Autodesk Fusion 360 part; units mm, degrees
(part 2 of 2)
  arc A148 (4.5, 28.5) -> (3.5, 27.5) centre (4.5, 27.5) ccw
  line L175 (1.7929, 170.8284) -> (15.7929, 156.8284)
  line L176 (17.5, 157.5355) -> (17.5, 159.833)
  line L177 (17.2071, 160.5402) -> (3.2071, 174.5402)
  line L178 (1.5, 173.833) -> (1.5, 171.5355)
  arc A149 (1.5, 171.5355) -> (1.7929, 170.8284) centre (2.5, 171.5355) ccw
  arc A150 (3.2071, 174.5402) -> (1.5, 173.833) centre (2.5, 173.833) ccw
  arc A151 (17.5, 159.833) -> (17.2071, 160.5402) centre (16.5, 159.833) ccw
  arc A152 (15.7929, 156.8284) -> (17.5, 157.5355) centre (16.5, 157.5355) ccw
  line L179 (2.3284, 9.7071) -> (8.7929, 16.1716)
  line L180 (10.5, 15.4645) -> (10.5, 9)
  line L181 (9.5, 8) -> (3.0355, 8)
  arc A153 (2.3284, 9.7071) -> (3.0355, 8) centre (3.0355, 9) ccw
  arc A154 (9.5, 8) -> (10.5, 9) centre (9.5, 9) ccw
  arc A155 (10.5, 15.4645) -> (8.7929, 16.1716) centre (9.5, 15.4645) ccw
  arc A156 (-23.9472, 177.9837) -> (-22.7624, 177.0888) centre (-22.951, 178.0708) ccw
  arc A157 (-24.2217, 193.0163) -> (-25.1674, 191.9304) centre (-24.1712, 192.0175) ccw
  arc A158 (19.6886, 185.2415) -> (20.4962, 186.3107) centre (19.5, 186.2235) ccw
  arc A159 (19.7989, 194.2803) -> (18.7522, 195.1918) centre (18.8028, 194.1931) ccw
  line L182 (-22.5614, 176.267) -> (-23.6581, 177.3637)
  point P0 (19.8308, 195.2464)
  point P1 (-25.2578, 192.9638)
  point P2 (-23.8633, 177.0247)
  point P3 (-87.3104, 78.3815)
  dimension "d191" = 1
  dimension "d192" = 7.5
  dimension "d193" = 1.5
  dimension "d194" = 27
  dimension "d195" = 24
  dimension "d196" = 35
  dimension "d199" = 1.5
  dimension "d200" = 2.5
  dimension "d201" = 5
  dimension "d202" = 2
  dimension "d203" = 0.4
  dimension "d204" = 1
  dimension "d205" = 30
  dimension "d206" = 0.2
  dimension "d207" = 5
  dimension "d209" = 2
  dimension "d210" = 3
  dimension "d211" = 1
  dimension "d212" = 20
  dimension "d214" = 20
  dimension "d215" = 180
  dimension "d216" = 90
  dimension "d217" = 5
  dimension "d225" = 2
  dimension "d228" = 2
  dimension "d229" = 1.5
  dimension "d230" = 45
  dimension "d233" = 10
  dimension "d234" = 12.7
  dimension "d235" = 3
  dimension "d237" = 20
  dimension "d240" = 2
  dimension "d241" = 2
  dimension "d242" = 2
  dimension "d243" = 16
  dimension "d245" = 45
  dimension "d246" = 20
  dimension "d247" = 20
  dimension "d249" = 90
  dimension "d250" = 5
  dimension "d251" = 5
  dimension "d252" = 3
  dimension "d253" = 5
  dimension "d287" = 20
  dimension "d288" = 2
  dimension "d296" = 5
  dimension "d297" = 2
  dimension "d299" = 60
  dimension "d300" = 2.5
  dimension "d301" = 1
  dimension "d303" = 360
  dimension "d306" = 7.5
  dimension "d307" = 5
  dimension "d309" = 30
  dimension "d310" = 1
  dimension "d311" = 20
  dimension "d312" = 3
  dimension "d313" = 1
  dimension "d314" = 3
  dimension "d315" = 1.5
  dimension "d316" = 1.5
  dimension "d317" = 1
  dimension "d318" = 1.5
  dimension "d319" = 3
  dimension "d320" = 1.5
  dimension "d321" = 1.5
  dimension "d322" = 3
  dimension "d323" = 1.5
  dimension "d324" = 1
  dimension "d325" = 1
  dimension "d326" = 3
  dimension "d327" = 1.5
  dimension "d328" = 1.5
  dimension "d329" = 3
  dimension "d330" = 3
  dimension "d331" = 3
  dimension "d332" = 3
  dimension "d333" = 1.5
  dimension "d334" = 1.5
  dimension "d335" = 1.5
  dimension "d336" = 1.5
  dimension "d337" = 1.5
  dimension "d338" = 1.5
  dimension "d339" = 1.5
  dimension "d340" = 1.5
  dimension "d341" = 1
  dimension "d342" = 1
  dimension "d343" = 3
  dimension "d344" = 1.5
  dimension "d345" = 1.5
  dimension "d346" = 1
  dimension "d347" = 1.5
  dimension "d348" = 3
  dimension "d349" = 3
  dimension "d350" = 1.5
  dimension "d351" = 1.5
  dimension "d352" = 3
  dimension "d353" = 1
  dimension "d354" = 3
  dimension "d355" = 3
  dimension "d356" = 1
  dimension "d357" = 1
  dimension "d358" = 1.5
  dimension "d359" = 45
  dimension "d360" = 1.5
  dimension "d361" = 3
  dimension "d362" = 1.5
  dimension "d363" = 1.5
  dimension "d364" = 3
  dimension "d365" = 1.5
  dimension "d366" = 1
  dimension "d369" = -20
  dimension "d370" = 0
  dimension "d371" = 1.5
  dimension "d372" = 3
  dimension "d373" = 1.5
  dimension "d374" = 1
  dimension "d375" = 1.5
  dimension "d376" = 3
  dimension "d377" = 3
  dimension "d378" = 3
  dimension "d379" = 1
  dimension "d380" = 1
  dimension "d381" = 3
  dimension "d382" = 3
  dimension "d383" = 3
  dimension "d390" = 1
  dimension "d391" = 100
  dimension "d392" = 14
  dimension "d393" = 8
  dimension "d394" = 20
  constraint vertical L0
  constraint perpendicular L0 L1
  constraint perpendicular L1 L2
  constraint perpendicular L2 L3
  constraint perpendicular L3 L4
  constraint perpendicular L4 L5
  constraint perpendicular L5 L6
  constraint perpendicular L0 L7
  constraint perpendicular L7 L8
  constraint perpendicular L0 L9
  constraint perpendicular L7 L10
  constraint perpendicular L0 L11
  constraint symmetric L2 L4 L12
  constraint symmetric L0 L6 L12
  constraint collinear origin L0.start L10.end
  constraint collinear origin L6.end L7.end
  constraint coincident L1 L5.end
  constraint perpendicular L1 L14
  constraint perpendicular L14 L15
  constraint tangent L14 A1
  constraint tangent L16 A1
  constraint tangent L14 A2
  constraint tangent L15 A2
  constraint equal A1 A2
  constraint tangent L15 A3
  constraint parallel L5 L17
  constraint perpendicular L5 L18
  constraint parallel L17 L20
  constraint perpendicular L17 L31
  constraint tangent L19 A4
  constraint tangent L17 A4
  constraint tangent L19 A5
  constraint tangent L20 A5
  constraint tangent L20 A6
  constraint tangent A6 L31
  constraint equal A5 A6
  constraint perpendicular L5 L21
  constraint tangent A4 L21
  constraint tangent L18 A7
  constraint perpendicular L13 L22
  constraint tangent L22 A7
  constraint horizontal L23
  constraint tangent A7 L23
  constraint coincident L6 L18.end
  constraint concentric A0 A8
  constraint coincident A8 L24.start
  constraint tangent A8 L24
  constraint perpendicular L24 L25
  constraint perpendicular L24 L27
  constraint tangent A0 L29
  constraint collinear L31 L32
  constraint perpendicular L22 L33
  constraint coincident origin L30
  constraint tangent L32 A9
  constraint tangent L33 A9
  constraint tangent L33 A10
  constraint tangent L30 A11
  constraint tangent L31 A11
  constraint concentric A0 A12
  constraint concentric A8 A13
  constraint vertical L36
  constraint parallel L29 L35
  constraint tangent L34 A14
  constraint tangent L36 A14
  constraint tangent L35 A15
  constraint tangent L36 A15
  constraint equal A14 A15
  constraint perpendicular L29 L37
  constraint tangent L29 A16
  constraint tangent L37 A17
  constraint tangent L28 A17
  constraint symmetric L24 P1 P2
  constraint vertical L38
  constraint tangent A3 L38
  constraint tangent A0 L39
  constraint tangent L37 A18
  constraint coincident L28 A17.start
  constraint perpendicular L38 L40
  constraint perpendicular L40 L41
  constraint tangent L40 A19
  constraint tangent L41 A19
  constraint coincident A20.centre A44.centre
  constraint coincident L32 A18.start
  constraint coincident A7.centre A21.centre
  constraint tangent L32 A21
  constraint coincident L32 A21.start
  constraint coincident L32.end A18.start
  constraint tangent L32 A18
  constraint coincident A0.centre A8.centre
  constraint tangent A22 A23
  constraint tangent L34 A23
  constraint tangent A22 A24
  constraint tangent L35 A24
  constraint equal A23 A24
  constraint horizontal L46
  constraint symmetric L43 L44 L46
  constraint parallel L43 L45
  constraint tangent L44 A27
  constraint tangent A25 A27
  constraint tangent A26 A28
  constraint tangent L44 A28
  constraint equal A27 A28
  constraint coincident P3 L43
  constraint coincident P3 A25
  constraint tangent A25 A29
  constraint tangent L43 A29
  constraint equal A27 A29
  constraint tangent A26 A30
  constraint tangent L43 A30
  constraint equal A27 A30
  constraint vertical L51
  constraint tangent L51 A44
  constraint tangent A43 A44
  constraint tangent A20 A43
  constraint tangent L51 A45
  constraint tangent L30 A45
  constraint collinear A20.centre A43.centre L52.end
  constraint perpendicular L12 L30
  constraint coincident L6.end L7
  constraint tangent L22 A46
  constraint tangent L7 A46
  constraint equal A9 A10
  constraint coincident A10.end A20.end
  constraint tangent A10 A20
  constraint horizontal L53
  constraint collinear A20.centre A10.end L53.end
  constraint midpoint L36 L54.start
  constraint coincident L39 L54.end
  constraint perpendicular L39 L54
  constraint coincident L34 L55.end
  constraint vertical L55
  constraint coincident L39 L56.end
  constraint perpendicular L39 L56
  constraint parallel L55 L57
  constraint coincident L34 L57.end
  constraint coincident L39 L58.end
  constraint perpendicular L39 L58
  constraint perpendicular L39 L60
  constraint vertical L61
  constraint tangent L59 A47
  constraint tangent L60 A47
  constraint tangent L60 A48
  constraint tangent L61 A48
  constraint equal A47 A48
  constraint tangent L59 A49
  constraint tangent L61 A49
  constraint equal A47 A49
  constraint parallel L39 L59
  constraint vertical L62
  constraint perpendicular L39 L64
  constraint perpendicular L63 L64
  constraint tangent L62 A50
  constraint tangent L64 A50
  constraint tangent L62 A51
  constraint tangent L63 A51
  constraint equal A50 A51
  constraint tangent L63 A52
  constraint tangent L64 A52
  constraint equal A50 A52
  constraint coincident L34 L65.start
  constraint coincident L39 L65.end
  constraint coincident L54 L65.start
  constraint parallel L12 L65
  constraint coincident L34 L66.end
  constraint perpendicular L34 L66
  constraint parallel L57 L69
  constraint perpendicular L39 L67
  constraint perpendicular L67 L68
  constraint tangent L67 A53
  constraint tangent L69 A53
  constraint tangent L68 A54
  constraint tangent L69 A54
  constraint equal A53 A54
  constraint tangent L67 A55
  constraint tangent L68 A55
  constraint equal A53 A55
  constraint perpendicular L39 L71
  constraint perpendicular L70 L71
  constraint parallel L57 L72
  constraint tangent L70 A56
  constraint tangent L72 A56
  constraint tangent L70 A57
  constraint tangent L71 A57
  constraint equal A56 A57
  constraint tangent L71 A58
  constraint tangent L72 A58
  constraint equal A56 A58
  constraint coincident L39 L73.end
  constraint vertical L73
  constraint coincident L34 L74.end
  constraint perpendicular L34 L74
  constraint coincident L40 L75.end
  constraint perpendicular L40 L75
  constraint perpendicular L78 L79
  constraint vertical L81
  constraint perpendicular L85 L87
  constraint perpendicular L83 L84
  constraint perpendicular L79 L80
  constraint perpendicular L34 L84
  constraint perpendicular L39 L87
  constraint perpendicular L39 L80
  constraint perpendicular L77 L78
  constraint parallel L65 L82
  constraint parallel L65 L86
  constraint parallel L73 L76
  constraint tangent L85 A59
  constraint tangent L87 A59
  constraint tangent L86 A60
  constraint tangent L87 A60
  constraint equal A59 A60
  constraint tangent L85 A61
  constraint tangent L86 A61
  constraint equal A59 A61
  constraint tangent L82 A62
  constraint tangent L84 A62
  constraint equal A59 A62
  constraint tangent L82 A63
  constraint tangent L83 A63
  constraint equal A59 A63
  constraint tangent L83 A64
  constraint tangent L84 A64
  constraint equal A59 A64
  constraint tangent L79 A65
  constraint tangent L80 A65
  constraint equal A59 A65
  constraint tangent L79 A66
  constraint tangent L81 A66
  constraint equal A59 A66
  constraint tangent L80 A67
  constraint tangent L81 A67
  constraint equal A59 A67
  constraint tangent L76 A68
  constraint tangent L77 A68
  constraint equal A59 A68
  constraint tangent L76 A69
  constraint tangent L78 A69
  constraint equal A59 A69
  constraint tangent L77 A70
  constraint tangent L78 A70
  constraint equal A59 A70
  constraint parallel L40 L90
  constraint parallel L74 L88
  constraint parallel L75 L89
  constraint tangent L90 A71
  constraint tangent L88 A71
  constraint tangent L89 A72
  constraint tangent L90 A72
  constraint equal A71 A72
  constraint tangent L88 A73
  constraint tangent L89 A73
  constraint equal A71 A73
  constraint parallel L75 L91
  constraint parallel L40 L93
  constraint parallel L34 L92
  constraint tangent L91 A74
  constraint tangent L93 A74
  constraint tangent L91 A75
  constraint tangent L92 A75
  constraint equal A74 A75
  constraint tangent L92 A76
  constraint tangent L93 A76
  constraint equal A74 A76
  constraint symmetric L46 L59.end L100.end
  constraint symmetric L46 L60.start L102.start
  constraint symmetric L46 A47 A85
  constraint symmetric L46 L60.end A84.start
  constraint symmetric L46 L61.start L101.start
  constraint symmetric L46 A48 A84
  constraint symmetric L46 L59.start A83.end
  constraint symmetric L46 L61.end A83.start
  constraint symmetric L46 A49 A83
  constraint symmetric L46 L62.start A86.end
  constraint symmetric L46 L64.end A86.start
  constraint symmetric L46 A50 A86
  constraint symmetric L46 L62.end L103.end
  constraint symmetric L46 L63.start L105.start
  constraint symmetric L46 A51 A88
  constraint symmetric L46 L63.end L105.end
  constraint symmetric L46 L64.start L104.start
  constraint symmetric L46 A52 A87
  constraint symmetric L46 L67.start A81.start
  constraint symmetric L46 L69.end L97.end
  constraint symmetric L46 A53 A81
  constraint symmetric L46 L68.end A80.end
  constraint symmetric L46 L69.start A80.start
  constraint symmetric L46 A54 A80
  constraint symmetric L46 L67.end L98.end
  constraint symmetric L46 L68.start L99.start
  constraint symmetric L46 A55 A82
  constraint symmetric L46 L70.start L94.start
  constraint symmetric L46 L72.end L96.end
  constraint symmetric L46 A56 A78
  constraint symmetric L46 L70.end L94.end
  constraint symmetric L46 L71.start L95.start
  constraint symmetric L46 A57 A79
  constraint symmetric L46 L71.end L95.end
  constraint symmetric L46 L72.start A77.end
  constraint symmetric L46 A58 A77
  constraint symmetric L46 L85.start A89.start
  constraint symmetric L46 L87.end A89.end
  constraint symmetric L46 A59 A89
  constraint symmetric L46 L86.end L108.end
  constraint symmetric L46 L87.start L107.start
  constraint symmetric L46 A60 A90
  constraint symmetric L46 L85.end L106.end
  constraint symmetric L46 L86.start L108.start
  constraint symmetric L46 A61 A91
  constraint symmetric L46 L82.start A92.end
  constraint symmetric L46 L84.end A92.start
  constraint symmetric L46 A62 A92
  constraint symmetric L46 L82.end L109.end
  constraint symmetric L46 L83.start L111.start
  constraint symmetric L46 A63 A94
  constraint symmetric L46 L83.end A93.start
  constraint symmetric L46 L84.start L110.start
  constraint symmetric L46 A64 A93
  constraint symmetric L46 L79.end L112.end
  constraint symmetric L46 L80.start L114.start
  constraint symmetric L46 A65 A97
  constraint symmetric L46 L79.start L112.start
  constraint symmetric L46 L81.end A95.start
  constraint symmetric L46 A66 A95
  constraint symmetric L46 L80.end A96.start
  constraint symmetric L46 L81.start L113.start
  constraint symmetric L46 A67 A96
  constraint symmetric L46 L76.end L115.end
  constraint symmetric L46 L77.start L117.start
  constraint symmetric L46 A68 A99
  constraint symmetric L46 L76.start L115.start
  constraint symmetric L46 L78.end L116.end
  constraint symmetric L46 A69 A98
  constraint symmetric L46 L77.end L117.end
  constraint symmetric L46 L78.start L116.start
  constraint symmetric L46 A70 A100
  constraint coincident L29 L118.start
  constraint coincident L35 L118.end
  constraint parallel L116 L118
  constraint perpendicular L119 L120
  constraint perpendicular L35 L119
  constraint tangent L119 A101
  constraint tangent L120 A101
  constraint tangent L119 A102
  constraint tangent L121 A102
  constraint equal A101 A102
  constraint tangent L120 A103
  constraint tangent L121 A103
  constraint equal A101 A103
  constraint symmetric L115 L118 L121
  constraint vertical L122
  constraint parallel L28 L123
  constraint parallel L121 L124
  constraint tangent L124 A104
  constraint tangent L123 A104
  constraint tangent L122 A105
  constraint tangent L124 A105
  constraint tangent L122 A106
  constraint tangent L123 A106
  constraint equal A105 A106
  constraint coincident L32 L125.end
  constraint perpendicular L32 L125
  constraint coincident L36 L126.end
  constraint coincident L32 L127.end
  constraint perpendicular L32 L127
  constraint coincident L36 L128.end
  constraint coincident L32 L129.end
  constraint perpendicular L32 L129
  constraint coincident L36 L130.end
  constraint parallel L126 L128
  constraint parallel L128 L130
  constraint coincident L32 L131.end
  constraint perpendicular L32 L131
  constraint parallel L130 L132
  constraint parallel L126 L136
  constraint parallel L126 L134
  constraint perpendicular L133 L135
  constraint perpendicular L137 L138
  constraint perpendicular L32 L138
  constraint perpendicular L36 L135
  constraint tangent L133 A107
  constraint tangent L134 A107
  constraint tangent L133 A108
  constraint tangent L135 A108
  constraint equal A107 A108
  constraint tangent L134 A109
  constraint tangent L135 A109
  constraint equal A107 A109
  constraint tangent L136 A110
  constraint tangent L137 A110
  constraint equal A107 A110
  constraint tangent L136 A111
  constraint tangent L138 A111
  constraint equal A107 A111
  constraint tangent L137 A112
  constraint tangent L138 A112
  constraint equal A107 A112
  constraint parallel L131 L151
  constraint perpendicular L151 L153
  constraint parallel L132 L152
  constraint tangent L151 A125
  constraint tangent L153 A125
  constraint tangent L152 A126
  constraint tangent L153 A126
  constraint equal A125 A126
  constraint tangent L151 A127
  constraint tangent L152 A127
  constraint equal A125 A127
  constraint symmetric L125 L133.end L154.end
  constraint symmetric L125 L134.start L156.start
  constraint symmetric L125 A107 A129
  constraint symmetric L125 L133.start L154.start
  constraint symmetric L125 L135.end A128.start
  constraint symmetric L125 A108 A128
  constraint symmetric L125 L134.end L156.end
  constraint symmetric L125 L135.start L155.start
  constraint symmetric L125 A109 A130
  constraint symmetric L125 L136.end L157.end
  constraint symmetric L125 L137.start A131.start
  constraint symmetric L125 A110 A131
  constraint symmetric L125 L136.start L157.start
  constraint symmetric L125 L138.end L159.end
  constraint symmetric L125 A111 A133
  constraint symmetric L125 L137.end L158.end
  constraint symmetric L125 L138.start A132.start
  constraint symmetric L125 A112 A132
  constraint symmetric L125 A113.start L160.start
  constraint symmetric L125 A113.end A134.start
  constraint symmetric L125 A113 A134
  constraint symmetric L125 A114.start A136.end
  constraint symmetric L125 A114.end L161.end
  constraint symmetric L125 A114 A136
  constraint symmetric L125 L140.start A135.end
  constraint symmetric L125 A115.end L160.end
  constraint symmetric L125 A115 A135
  constraint symmetric L125 L142.start A137.start
  constraint symmetric L125 L142.end L164.end
  constraint symmetric L125 A116.start L163.end
  constraint symmetric L125 A116 A137
  constraint symmetric L125 L143.start L163.start
  constraint symmetric L125 L144.start A138.start
  constraint symmetric L125 L144.end L165.end
  constraint symmetric L125 A117 A139
  constraint symmetric L125 A118 A138
  constraint symmetric L125 A119.start L167.start
  constraint symmetric L125 A119.end L166.end
  constraint symmetric L125 A119 A142
  constraint symmetric L125 A120.start A140.end
  constraint symmetric L125 A120.end A140.start
  constraint symmetric L125 A120 A140
  constraint symmetric L125 L146.start A141.end
  constraint symmetric L125 A121.end A141.start
  constraint symmetric L125 A121 A141
  constraint symmetric L125 L148.start A143.start
  constraint symmetric L125 L148.end L170.end
  constraint symmetric L125 A122.start A143.end
  constraint symmetric L125 A122 A143
  constraint symmetric L125 L149.start L169.start
  constraint symmetric L125 L150.start A144.start
  constraint symmetric L125 L150.end L171.end
  constraint symmetric L125 A123 A145
  constraint symmetric L125 A124 A144
  constraint symmetric L125 L151.start L173.start
  constraint symmetric L125 L153.end L174.end
  constraint symmetric L125 A125 A148
  constraint symmetric L125 L152.end L172.end
  constraint symmetric L125 L153.start L174.start
  constraint symmetric L125 A126 A147
  constraint symmetric L125 L151.end A146.end
  constraint symmetric L125 L152.start L172.start
  constraint symmetric L125 A127 A146
  constraint vertical L176
  constraint parallel L175 L177
  constraint perpendicular L131 L178
  constraint parallel L132 L175
  constraint tangent L175 A149
  constraint tangent L178 A149
  constraint tangent L177 A150
  constraint tangent L178 A150
  constraint equal A149 A150
  constraint tangent L176 A151
  constraint tangent L177 A151
  constraint equal A149 A151
  constraint tangent L175 A152
  constraint tangent L176 A152
  constraint equal A149 A152
  constraint tangent L179 A153
  constraint tangent L181 A153
  constraint tangent L180 A154
  constraint tangent L181 A154
  constraint equal A153 A154
  constraint tangent L179 A155
  constraint tangent L180 A155
  constraint equal A153 A155
  constraint parallel L172 L179
  constraint parallel L40 L181
  constraint parallel L12 L180
  constraint tangent L27 A156
  constraint tangent L28 A156
  constraint coincident P1 L26
  constraint coincident P1 L27
  constraint tangent L26 A157
  constraint tangent L27 A157
  constraint equal A156 A157
  constraint tangent L25 A158
  constraint tangent L28 A158
  constraint equal A156 A158
  constraint coincident P0 L26
  constraint tangent L25 A159
  constraint tangent L26 A159
  constraint equal A156 A159
  constraint coincident A156 L182.end
  constraint tangent A16 L182
  constraint tangent A156 L182
  constraint perpendicular L29 L182
  constraint tangent L32 A158
  measures "d191" distance of L1 L11
  measures "d192" distance of L3 L13
  measures "d193" distance of L3 L9
  measures "d194" distance of L2 L4
  measures "d195" distance of L8 L10
  measures "d196" distance of L0 L6
  measures "d199" radius of A1
  measures "d200" distance of L0 L14
  measures "d201" distance of L15 L16
  measures "d202" radius of A3
  measures "d203" radius of A4
  measures "d204" radius of A5
  measures "d205" angle of L4 L19
  measures "d206" distance of L5 L17
  measures "d207" distance of L5 L20
  measures "d209" distance of L18 L21
  measures "d210" distance of L18 L31
  measures "d211" diameter of A7
  measures "d212" distance of L7 L23
  measures "d214" radius of A0
  measures "d215" diameter of A8
  measures "d216" distance of L11 A0.centre
  measures "d217" angle of L13 L24
  measures "d225" radius of A9
  measures "d228" radius of A11
  measures "d229" distance of L0 A3.centre
  measures "d230" distance of L25 L27
  measures "d233" distance of L30 A20.centre
  measures "d234" diameter of A12
  measures "d235" diameter of A13
  measures "d237" distance of L29 L35
  measures "d240" radius of A14
  measures "d241" radius of A16
  measures "d242" radius of A17
  measures "d243" distance of P1 P2
  measures "d245" angle of L13 L39
  measures "d246" distance of L34 L39
  measures "d247" distance of L32 L36
  measures "d249" angle of L29 L39
  measures "d250" distance of L11 L38.end
  measures "d251" radius of A18
  measures "d252" distance of L22 L41
  measures "d253" radius of A19
  measures "d287" radius of A22
  measures "d288" radius of A23
  measures "d296" distance of L39 P3
  measures "d297" distance of A12 A26
  measures "d299" angle of L45 L46
  measures "d300" distance of L43 L45
  measures "d301" radius of A27
  measures "d306" radius of A44
  measures "d307" distance of A20 A44
  measures "d309" angle of L30 L52
  measures "d310" radius of A46
  measures "d311" distance of L32 A20.centre
  measures "d312" radius of A45
  measures "d313" radius of A47
  measures "d314" distance of L39 L59
  measures "d315" distance of L56 L60
  measures "d316" distance of L55 L61
  measures "d317" radius of A50
  measures "d318" distance of L55 L62
  measures "d319" distance of L34 L63
  measures "d320" distance of L54 L64
  measures "d321" distance of L56 L67
  measures "d322" distance of L34 L68
  measures "d323" distance of L57 L69
  measures "d324" radius of A53
  measures "d325" radius of A56
  measures "d326" distance of L39 L70
  measures "d327" distance of L57 L72
  measures "d328" distance of L58 L71
  measures "d329" distance of L39 L85
  measures "d330" distance of L39 L79
  measures "d331" distance of L34 L77
  measures "d332" distance of L34 L83
  measures "d333" distance of L66 L84
  measures "d334" distance of L66 L80
  measures "d335" distance of L73 L81
  measures "d336" distance of L73 L76
  measures "d337" distance of L74 L78
  measures "d338" distance of L65 L82
  measures "d339" distance of L65 L86
  measures "d340" distance of L54 L87
  measures "d341" radius of A59
  measures "d342" radius of A71
  measures "d343" distance of L40 L90
  measures "d344" distance of L74 L88
  measures "d345" distance of L75 L89
  measures "d346" radius of A74
  measures "d347" distance of L75 L91
  measures "d348" distance of L34 L92
  measures "d349" distance of L40 L93
  measures "d350" distance of L116 L118
  measures "d351" distance of L118 L119
  measures "d352" distance of L35 L120
  measures "d353" radius of A101
  measures "d354" distance of L121 L124
  measures "d355" distance of L28 L123
  measures "d356" radius of A104
  measures "d357" radius of A105
  measures "d358" distance of L12 L122
  measures "d359" angle of L125 L126
  measures "d360" distance of L125 L135
  measures "d361" distance of L36 L133
  measures "d362" distance of L126 L134
  measures "d363" distance of L126 L136
  measures "d364" distance of L32 L137
  measures "d365" distance of L127 L138
  measures "d366" radius of A107
  measures "d371" distance of L131 L151
  measures "d372" distance of L36 L153
  measures "d373" distance of L132 L152
  measures "d374" radius of A125
  measures "d375" distance of L132 L175
  measures "d376" distance of L32 L176
  measures "d377" distance of L37 L177
  measures "d378" distance of L122 L178
  measures "d379" radius of A149
  measures "d380" radius of A153
  measures "d381" distance of L40 L181
  measures "d382" distance of L172 L179
  measures "d383" distance of L41 L180
  measures "d390" radius of A156
  measures "d391" distance of A0.centre L182
  measures "d392" distance of A156.centre A157.centre
  measures "d393" distance of A158.centre A159.centre
  measures "d394" distance of L37 L182
extrude "押し出し4" add sketch "スケッチ6" along normal blind 16.5 separate body contours L0 L1 L6 L7 L11 L13 L14 L15 L16 A1 A2 A3 L17 L18 L19 L20 A4 A5 A6 L22 A7 L30 L31 L32 L33 A9 A10 A11 L38 L40 L41 A19 L42 A20 A21 L51 A43 A44 A45 A46 | L24 L25 L26 L27 A157 A159 | L24 L25 L27 L28 A156 A158 makes body 2 at (26.1667, 2.6667, 0) makes body 3 at (-8.6121, 179.8063, 5.5)
extrude "押し出し5" add sketch "スケッチ6" along normal blind 3 contours L39 L40 L74 L75 | A8 L39 L73 A66 | A8 L34 L73 L74 L76 L77 L78 A69 A70 | L12 L34 A14 L40 L75 | A8 L39 L66 L73 L79 L80 L81 A65 A66 A67 | A8 L34 L73 L76 L77 A68 | L12 A8 L32 L36 A14 L40 L41 A19 A21 L125 L155 L156 A130 L157 A131 L158 A132 L159 L161 A136 L162 | A8 A66 | L39 L54 L65 | L34 L65 L66 | A8 L29 L35 A95 L115 L116 A98 L117 A100 L118 | A0 A8 L29 L34 L35 L39 A22 A23 A24 L56 L57 L58 L112 A95 L113 A96 L114 A97 L115 L117 A99 | L34 L54 L55 | L39 L55 L56 | A8 L36 L125 L154 A128 L155 L156 A129 L157 L159 A133 L160 A134 A135 L161 L162 | A8 A95 | L28 L29 L32 L35 L36 A15 L37 A16 A17 A18 L118 L131 A156 L182 | L39 L57 L58 | A8 L36 L125 L126 L133 L134 L135 A107 A108 | A8 L126 L127 L136 L138 A111 | A8 L36 L127 L128 A113 L139 L140 A115 L141 | A8 L125 L126 L134 L135 A109 | A8 L128 L129 | A8 L36 L129 | A8 L32 L126 L127 L136 L137 L138 A110 A112 | A8 L127 L128 A114 L139 L140 | A8 L36 L129 L130 | A8 L32 L128 L129 | L32 L130 L131 | A12 bodies 2 3
ref_plane "作業平面2" through (0, 90, 0) normal (0, 1, 0) x (0, 0, 1)
sketch "スケッチ7" plane through (0, 90, 0) normal (0, 1, 0) x (1, 0, 0)
  line L0 (-71.3657, 0) -> (-71.3657, -14.3)
  line L1 (-71.3657, -16.5) -> (-72.5657, -16.5)
  line L2 (-72.9657, -16.1) -> (-72.9657, -5.75)
  line L3 (-71.3657, -16.5) -> (-70.5657, -15.7)
  line L4 (-71.3657, -16.5) -> (-70.7411, -16.5) construction
  line L5 (-70.5657, -15.7) -> (-70.5657, -15.1)
  line L6 (-70.5657, -15.1) -> (-71.3657, -14.3)
  line L7 (-77.7157, 1.5) -> (-77.7157, -4.5)
  line L8 (-72.9657, 0) -> (-71.3657, 0)
  line L9 (-72.5657, -16.5) -> (-72.9657, -16.1)
  line L10 (-167.7157, 0) -> (12.2843, 0)
  line L11 (-72.9657, -5.75) -> (-75.7157, -3)
  line L12 (-75.7157, -3) -> (-75.7157, 0)
  point P0 (-77.7157, 0)
  dimension "d262" = 45
  dimension "d263" = 45
  dimension "d264" = 6.35
  dimension "d265" = 1.6
  dimension "d268" = 16.5
  dimension "d269" = 0.4
  dimension "d270" = 0.4
  dimension "d271" = 0.8
  dimension "d272" = 0.6
  dimension "d395" = 2
  dimension "d397" = 3
  dimension "d398" = 45
  constraint vertical L0
  constraint perpendicular L0 L1
  constraint perpendicular L1 L2
  constraint horizontal L4
  constraint perpendicular L1 L5
  constraint perpendicular L0 L8
  constraint coincident L8 P0
  constraint collinear L0.start L1.start L0.end
  constraint coincident L10 L12.end
  constraint perpendicular L10 L12
  measures "d262" angle of L3 L4
  measures "d263" angle of L5 L6
  measures "d264" distance of L0 L7
  measures "d265" distance of L0 L2
  measures "d268" distance of L1 L10
  measures "d269" horizontal distance of L1.end L2.start
  measures "d270" vertical distance of L1.end L2.start
  measures "d271" horizontal distance of L3.end L0.end
  measures "d272" distance of L3.end L5.end
  measures "d395" distance of L7 L12
  measures "d397" distance of L11.end L12.end
  measures "d398" angle of L10 L11
revolve "回転2" add sketch "スケッチ7" angle 360 about axis through (-77.7157, 90, -1.5) along (0, 0, 1) bodies 2
sketch "スケッチ8" plane through (0, 0, 16.5) normal (0, 0, 1) x (-1, 0, 0)
  circle A0 centre (77.7157, -90) radius 6.35
  circle A1 centre (77.7157, -90) radius 5.15
  line L0 (77.7157, -90) -> (76.7157, -90)
  line L1 (76.7157, -91) -> (68.7157, -91)
  line L2 (68.7157, -91) -> (68.7157, -89)
  line L3 (68.7157, -89) -> (76.7157, -89)
  line L4 (76.7157, -89) -> (76.7157, -91)
  line L5 (79.0818, -90.366) -> (83.0818, -97.2942)
  line L6 (77.3497, -91.366) -> (79.0818, -90.366)
  line L7 (83.0818, -97.2942) -> (81.3497, -98.2942)
  line L8 (81.3497, -98.2942) -> (77.3497, -91.366)
  line L9 (77.3497, -88.634) -> (81.3497, -81.7058)
  line L10 (79.0818, -89.634) -> (77.3497, -88.634)
  line L11 (81.3497, -81.7058) -> (83.0818, -82.7058)
  line L12 (83.0818, -82.7058) -> (79.0818, -89.634)
  dimension "d274" = 1
  dimension "d275" = 2
  dimension "d276" = 8
  dimension "d278" = 360
  constraint coincident A0.centre A1.centre
  constraint horizontal L0
  constraint horizontal L1
  constraint vertical L2
  constraint horizontal L3
  constraint vertical L4
  constraint symmetric L0 L1 L3
  constraint coincident L0.end L4
  measures "d274" distance of A0.centre L0.end
  measures "d275" distance of L1 L3
  measures "d276" distance of L2 L4
extrude "押し出し6" cut sketch "スケッチ8" against normal blind 13.5 contours A0 A1 L9 L12 | A0 L9 L11 L12 | A0 L5 L7 L8 | A0 A1 L5 L8 | A1 L9 L10 L12 | A1 L5 L6 L8 | A0 A1 L1 L3 | A0 L1 L2 L3 | A1 L1 L3 L4 bodies 2
sketch "スケッチ9" plane through (36.5168, 3.1948, 0) normal (0.996195, 0.087156, 0) x (-0.087156, 0.996195, 0)
  line L0 (183.8154, 0) -> (191.8154, 0)
  line L1 (191.8154, 16.5) -> (183.8154, 16.5)
  line L2 (186.3154, 14.25) -> (189.3154, 14.25)
  line L3 (189.3154, 14.25) -> (189.3154, 5.25)
  line L4 (189.3154, 5.25) -> (186.3154, 5.25)
  line L5 (186.3154, 5.25) -> (186.3154, 14.25)
  line L6 (186.3154, 9.75) -> (189.3154, 9.75)
  line L7 (187.8154, 14.25) -> (187.8154, 5.25)
  line L8 (191.8154, 0) -> (191.8154, 16.5)
  line L9 (183.8154, 16.5) -> (183.8154, 0)
  dimension "d289" = 6.75
  dimension "d290" = 9
  dimension "d291" = 3
  constraint horizontal L2
  constraint vertical L3
  constraint horizontal L4
  constraint vertical L5
  constraint midpoint L5 L6.start
  constraint midpoint L3 L6.end
  constraint midpoint L2 L7.start
  constraint midpoint L4 L7.end
  constraint symmetric L7 L8 L9
  measures "d289" distance of L1 L6
  measures "d290" distance of L2 L4
  measures "d291" distance of L3 L5
sketch "スケッチ10" plane through (-8.312, -0.7272, 0) normal (-0.996195, -0.087156, 0) x (0.087156, -0.996195, 0)
  line L0 (-193.3935, 0) -> (-179.3935, 0)
  line L1 (-179.3935, 16.5) -> (-193.3935, 16.5)
  line L2 (-190.3935, 14.75) -> (-185.3935, 14.75)
  line L3 (-185.3935, 14.75) -> (-185.3935, 4.75)
  line L4 (-185.3935, 4.75) -> (-190.3935, 4.75)
  line L5 (-190.3935, 4.75) -> (-190.3935, 14.75)
  line L6 (-187.8935, 14.75) -> (-187.8935, 4.75)
  line L7 (-190.3935, 9.75) -> (-185.3935, 9.75)
  line L8 (-179.3935, 0) -> (-179.3935, 16.5)
  line L9 (-193.3935, 16.5) -> (-193.3935, 0)
  dimension "d292" = 6.75
  dimension "d293" = 10
  dimension "d294" = 5
  dimension "d407" = 3
  constraint horizontal L2
  constraint vertical L3
  constraint horizontal L4
  constraint vertical L5
  constraint midpoint L2 L6.start
  constraint midpoint L4 L6.end
  constraint midpoint L5 L7.start
  constraint midpoint L3 L7.end
  measures "d292" distance of L1 L7
  measures "d293" distance of L2 L4
  measures "d294" distance of L3 L5
  measures "d407" distance of L5 L9
loft "ロフト2" cut profiles "スケッチ10", "スケッチ9" section 1 contours L2 L5 L6 L7 | L2 L3 L6 L7 | L4 L5 L6 L7 | L3 L4 L6 L7 section 2 contours L2 L5 L6 L7 | L2 L3 L6 L7 | L4 L5 L6 L7 | L3 L4 L6 L7 bodies 2
fillet "フィレット4" radius 2 2 edges at (-24.9059, 188.9418, 9.75) (-24.4701, 183.9608, 9.75) on bodies 2
chamfer "面取り4" distance 0.8 angle 45 6 edges at (-80.5825, 92.9653, 3) (-80.5825, 87.0347, 3) (-78.8504, 86.0347, 3) (-73.7143, 89, 3) (-73.7143, 91, 3) (-78.8504, 93.9653, 3) on bodies 2
chamfer "面取り5" distance 1 angle 45 2 edges at (-9.3071, 179.6729, 3) (-23.2444, 177.1148, 3) on bodies 2
hidden bodies 2
equation "d67 = 6.35 mm + 3 mm"
equation "d143 = 6.35 mm + 2.5 mm"
